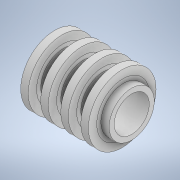
# Autodesk Inventor part: Демфер пальца
Saved by Autodesk Inventor 2021 (Build 250183000, 183)
## iProperties
Created: 2023-04-15
Part Number: Демфер пальца
Material: Типовые
Document SubType Name: Modeling
Designer: gdevc
Density: 1 g/cm^3
Appearance: По умолчанию
Author: gdevc
Autodesk Inventor part; units mm, degrees
ref_plane "YZ Plane" through (0, 0, 0) normal (1, 0, 0) x (0, 1, 0)
ref_plane "XZ Plane" through (0, 0, 0) normal (0, 1, 0) x (-1, 0, 0)
ref_plane "XY Plane" through (0, 0, 0) normal (0, 0, 1) x (1, 0, 0)
sketch "Эскиз1" plane through (0, 0, 0) normal (0, 0, 1) x (1, 0, 0)
  line L0 (0, 0) -> (32, 0)
  line L1 (0, 7) -> (33.2977, 7)
  line L2 (4, 13.5) -> (2.5, 13.5)
  line L3 (2.5, 13.5) -> (2.1775, 10.5)
  line L4 (2.1775, 10.5) -> (1.9988, 9)
  line L5 (1.9988, 9) -> (0, 9)
  line L6 (0, 9) -> (0, 7)
  line L7 (4, 13.5) -> (4, 8.1664)
  line L8 (4, 13.5) -> (5.5, 13.5)
  line L9 (5.5, 13.5) -> (5.8225, 10.5)
  line L10 (5.8225, 10.5) -> (6.0012, 9)
  line L11 (6.0012, 9) -> (8, 9)
  line L12 (13.5, 13.5) -> (13.8225, 10.5)
  line L13 (13.8225, 10.5) -> (14.0012, 9)
  line L14 (14.0012, 9) -> (16, 9)
  line L15 (10.1775, 10.5) -> (9.9988, 9)
  line L16 (10.5, 13.5) -> (10.1775, 10.5)
  line L17 (9.9988, 9) -> (8, 9)
  line L18 (16, 9) -> (16, 13.7658)
  line L19 (28, 13.5) -> (29.5, 13.5)
  line L20 (29.5, 13.5) -> (29.8225, 10.5)
  line L21 (29.8225, 10.5) -> (30.0012, 9)
  line L22 (26.1775, 10.5) -> (25.9988, 9)
  line L23 (26.5, 13.5) -> (26.1775, 10.5)
  line L24 (28, 13.5) -> (26.5, 13.5)
  line L25 (25.9988, 9) -> (24, 9)
  line L26 (17.9988, 9) -> (16, 9)
  line L27 (18.1775, 10.5) -> (17.9988, 9)
  line L28 (18.5, 13.5) -> (18.1775, 10.5)
  line L29 (21.5, 13.5) -> (21.8225, 10.5)
  line L30 (21.8225, 10.5) -> (22.0012, 9)
  line L31 (22.0012, 9) -> (24, 9)
  line L32 (30.0012, 9) -> (33.2977, 9)
  line L33 (33.2977, 9) -> (33.2977, 7)
  line L34 (10.5, 13.5) -> (13.5, 13.5)
  line L35 (18.5, 13.5) -> (21.5, 13.5)
  point P0 (1.5, 8.1664)
  dimension "d14" = 32
  dimension "d15" = 14
  dimension "d16" = 27
  dimension "d20" = 4
  dimension "d22" = 3
  dimension "d33" = 1.5
  dimension "d35" = 2
  constraints: 72 end point, 18 symmetric about line, 6 horizontal, 2 perpendicular, 2 vertical, 1 collinear
  measures "d14" distance of L0.start L0.end
  measures "d15" diameter of L1 L0
  measures "d16" diameter of L2.start L0
  measures "d20" horizontal distance of L0.start L2.start
  measures "d22" vertical distance of L3.end L2.start
  measures "d33" distance of L2.start L2.end
  measures "d35" distance between parallel lines of L1 L5
revolve "Вращение1" add sketch "Эскиз1" angle 360 about axis through (0, 0, 0) along (1, 0, 0)
